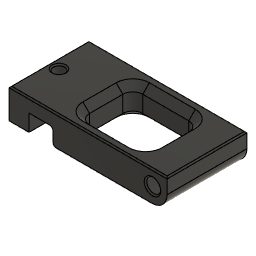
bowen_retainer (Autodesk Fusion 360 design; units mm, degrees)
Autodesk Fusion 360 part; units mm, degrees
sketch "Sketch1" plane through (0, 0, 0) normal (0, 1, 0) x (1, 0, 0) in component "bowen_retainer"
  line L0 (-24, -4) -> (23.5, -4)
  line L1 (23.5, -4) -> (23.5, 5)
  line L2 (23.5, 5) -> (-10.809, 5)
  line L3 (-10.809, 5) -> (-10.809, 0)
  line L4 (-10.809, 0) -> (-18, 0)
  line L5 (-18, 0) -> (-18, 6)
  line L6 (-18, 6) -> (-24, 6)
  line L7 (-24, 6) -> (-24, -4)
  circle A0 centre (19.1, 0.5) radius 2.1
  line L8 (23.5, 0.5) -> (19.1, 0.5) construction
  point P0 (23.5, 0.5)
  dimension "d17" = 47.5
  dimension "d18" = 6
  dimension "d19" = 6
  dimension "d22" = 9
  dimension "d23" = 4.2
  dimension "d24" = 4.4
  constraint horizontal L0
  constraint perpendicular L0 L1
  constraint perpendicular L1 L2
  constraint perpendicular L2 L3
  constraint perpendicular L3 L4
  constraint perpendicular L4 L5
  constraint perpendicular L5 L6
  constraint perpendicular L0 L7
  constraint midpoint L1 P0
  constraint coincident P0 L8.start
  constraint coincident A0.centre L8.end
  constraint perpendicular L1 L8
  measures "d17" distance of L0.start L0.end
  measures "d18" distance of L5.end L6.end
  measures "d19" distance of L4.end L5.end
  measures "d22" distance of L0.end L1.end
  measures "d23" diameter of A0
  measures "d24" distance of L1 A0.centre
extrude "Extrude1" add sketch "Sketch1" along normal mid plane 24 in component "bowen_retainer"
sketch "Sketch2" plane through (0, 0, 4) normal (0, 0, 1) x (-1, 0, 0) in component "bowen_retainer"
  line L0 (-23.5, 12) -> (-23.5, -12)
  line L1 (-23.5, -12) -> (24, -12)
  line L2 (24, -12) -> (24, 12)
  line L3 (24, 12) -> (-23.5, 12)
  circle A0 centre (21, 0) radius 1.7
  line L4 (24, 12) -> (24, -12)
  line L5 (24, -12) -> (18, -12)
  line L6 (18, -12) -> (18, 12)
  line L7 (18, 12) -> (24, 12)
  line L8 (24, -12) -> (18, 12) construction
  line L9 (24, 12) -> (18, -12) construction
  line L10 (6.809, -8) -> (-13, -8)
  line L11 (-13, -8) -> (-13, 8)
  line L12 (-13, 8) -> (6.809, 8)
  line L13 (6.809, 8) -> (6.809, -8)
  line L14 (10.809, 12) -> (10.809, -12)
  line L15 (10.809, -12) -> (-23.5, -12)
  line L16 (-23.5, -12) -> (-23.5, 12)
  line L17 (-23.5, 12) -> (10.809, 12)
  point P0 (21, 0)
  dimension "d27" = 3.4
  dimension "d28" = 4
  dimension "d29" = 4
  dimension "d30" = 10.5
  dimension "d31" = 4
  constraint coincident L1.end L2.start
  constraint coincident L6.end L7.start
  constraint coincident L2.end L3.start
  constraint coincident L5.end L6.start
  constraint midpoint L9 P0
  constraint coincident P0 A0.centre
  constraint horizontal L10
  constraint vertical L11
  constraint horizontal L12
  constraint vertical L13
  measures "d27" diameter of A0
  measures "d28" distance of L1 L10
  measures "d29" distance of L3 L12
  measures "d30" distance of L0 L11
  measures "d31" distance of L13 L14
extrude "Extrude2" cut sketch "Sketch2" against normal through all contours A0 | L10 L11 L12 L13 in component "bowen_retainer"
sketch "Sketch3" plane through (-24, 0, 0) normal (-1, 0, 0) x (0, -1, 0) in component "bowen_retainer"
  line L0 (12, 4) -> (-12, 4)
  line L1 (-12, 4) -> (-12, -6)
  line L2 (-12, -6) -> (12, -6)
  line L3 (12, -6) -> (12, 4)
  line L4 (-6, -6) -> (6, -6)
  line L5 (6, -6) -> (6, 0)
  line L6 (6, 0) -> (-6, 0)
  line L7 (-6, 0) -> (-6, -6)
  line L8 (12, 0) -> (-12, 0)
  line L9 (-12, 0) -> (-12, -5)
  line L10 (-12, -5) -> (12, -5)
  line L11 (12, -5) -> (12, 0)
  dimension "d33" = 6
  constraint horizontal L4
  constraint vertical L5
  constraint horizontal L6
  constraint vertical L7
  constraint coincident L2 L4.start
  constraint collinear L6 L8
  constraint midpoint L6 L8
  measures "d33" distance of L1 L7
extrude "Extrude3" cut sketch "Sketch3" against normal up to surface (6 mm away) contours L5 L6 L7 L8 L10 | L2 L4 L5 L7 L10 in component "bowen_retainer"
fillet "Fillet1" radius 4.5 1 edges at (23.5, 0, -5) in component "bowen_retainer"
fillet "Fillet2" radius 3 4 edges at (-6.809, 8, -0.5) (13, 8, -0.5) (13, -8, -0.5) (-6.809, -8, -0.5) in component "bowen_retainer"
chamfer "Chamfer1" distance 2 angle 45 16 edges at (-5.9304, 7.1213, 4) (-6.809, 0, 4) (-5.9304, -7.1213, 4) (3.0955, -8, 4) (12.1213, -7.1213, 4) (13, 0, 4) (12.1213, 7.1213, 4) (3.0955, 8, 4) (-6.809, 0, -5) (-5.9304, -7.1213, -5) (3.0955, -8, -5) (12.1213, -7.1213, -5) (13, 0, -5) (12.1213, 7.1213, -5) (3.0955, 8, -5) (-5.9304, 7.1213, -5) in component "bowen_retainer"
fillet "Fillet3" radius 1 2 edges at (-10.809, 0, 0) (-10.809, 0, -5) in component "bowen_retainer"
chamfer "Chamfer2" distance 1 angle 45 2 edges at (-24, 9, -6) (-21, 12, -6) 2 faces at (-20, 8, -6) (-20, -8, -6) in component "bowen_retainer"
chamfer "Chamfer3" distance 0.4 angle 45 7 edges at (-19.415, -0.6147, 4) (17.1421, -12, 0.2594) (17.1421, 12, -1.2594) (-0.25, 12, 4) (23.5, 0, 4) (-0.25, -12, 4) (-24, 0, 4) in component "bowen_retainer"
component "bowen_retainer" placed x (1, 0, 0) y (0, 1, 0) z (0, 0, 1) at (0, 0, 0)
equation "ptfe_tube_od = 4 mm"
equation "tolerance = 0.2 mm"
equation "extrusion_width = 20 mm"
equation "width = 24 mm"
equation "length = 47.5 mm"
equation "arm_width = 4 mm"
equation "extrusion_slot_width = 6 mm"
equation "d17 = length"
equation "d18 = extrusion_slot_width"
equation "d19 = extrusion_slot_depth"
equation "extrusion_slot_depth = 6 mm"
equation "depth = 9 mm"
equation "d22 = depth"
equation "d23 = ptfe_tube_od + tolerance"
equation "d25 = width"
equation "d28 = arm_width"
equation "d29 = arm_width"
equation "d33 = extrusion_slot_depth"
